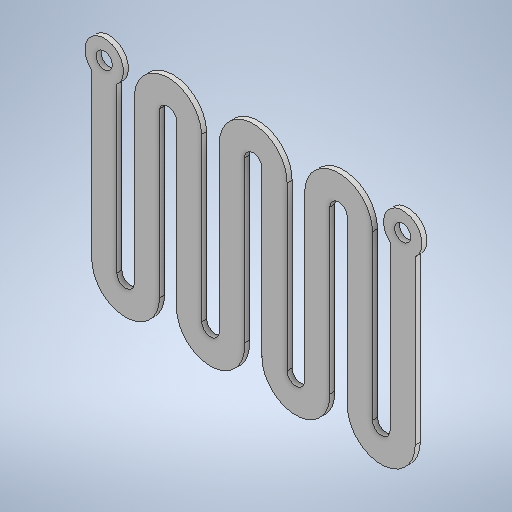
# Autodesk Inventor part: sensor2
Saved by Autodesk Inventor 2025.2 (Build 292293000, 293)
## iProperties
Created: 2025-01-22
Part Number: sensor2
Material: Generic
Document SubType Name: Modeling
Designer: Tony Dias
Density: 1 g/cm^3
Appearance: Default
Author: Tony Dias
Autodesk Inventor part; units mm, degrees
ref_plane "YZ Plane" through (0, 0, 0) normal (1, 0, 0) x (0, 1, 0)
ref_plane "XZ Plane" through (0, 0, 0) normal (0, 1, 0) x (-1, 0, 0)
ref_plane "XY Plane" through (0, 0, 0) normal (0, 0, 1) x (1, 0, 0)
sketch "Sketch1" plane through (0, 0, 0) normal (0, 0, 1) x (1, 0, 0)
  circle A0 centre (-59.5535, 47.2459) radius 7.653
  line L0 (-64.5524, 41.4512) -> (-64.5524, -23.1778)
  line L1 (-54.5526, 41.4529) -> (-54.5526, -23.5479)
  arc A1 (-54.5526, -23.5479) -> (-47.5527, -23.4962) centre (-51.0525, -23.5479) ccw
  line L2 (-47.5527, -23.4962) -> (-47.5527, 41.452)
  line L3 (-37.5474, 41.5644) -> (-37.5474, -23.5532)
  arc A2 (-64.5524, -23.1778) -> (-37.5474, -23.5515) centre (-51.0525, -23.5479) ccw
  arc A3 (-30.8632, 41.7144) -> (-37.5474, 41.5644) centre (-34.182, 40.6024) ccw
  line L4 (-30.8632, 41.7144) -> (-30.8632, -23.4297)
  line L5 (-20.7948, 41.1318) -> (-20.7948, -23.4297)
  arc A4 (-20.7947, 41.1274) -> (-47.5527, 41.452) centre (-34.182, 40.6024) ccw
  line L6 (-13.7626, 41.5703) -> (-13.7626, -23.4297)
  arc A5 (-20.7948, -23.4297) -> (-13.7626, -23.4297) centre (-17.2787, -23.4297) ccw
  line L7 (-3.7454, 41.5703) -> (-3.7454, -22.2525)
  arc A6 (-30.8632, -23.4297) -> (-3.7454, -22.2525) centre (-17.2787, -23.4297) ccw
  line L8 (3.17, 41.5703) -> (3.17, -23.406)
  line L9 (13.1831, 41.5703) -> (13.1831, -23.4297)
  arc A7 (3.17, 41.5703) -> (-3.7454, 41.5703) centre (-0.2877, 41.5703) ccw
  arc A8 (13.1831, 41.2384) -> (-13.7626, 41.5703) centre (-0.2877, 41.5703) ccw
  line L10 (20.1776, 41.5703) -> (20.1776, -23.4297)
  arc A9 (13.1831, -23.4297) -> (20.1776, -23.4297) centre (16.6804, -23.4297) ccw
  line L11 (30.1804, -22.8989) -> (30.1804, 41.5703)
  arc A10 (3.17, -23.406) -> (30.1804, -22.8989) centre (16.6804, -23.4297) ccw
  line L12 (37.1748, 41.5703) -> (37.1748, -23.4297)
  line L13 (47.1776, 41.5703) -> (47.1776, -23.4297)
  arc A11 (37.1748, 41.5703) -> (30.1804, 41.5703) centre (33.6776, 41.5703) ccw
  arc A12 (47.1776, 41.5703) -> (20.1776, 41.5703) centre (33.6776, 41.5703) ccw
  circle A13 centre (-59.5535, 47.2459) radius 3.25
  line L14 (54.172, -23.4297) -> (54.172, 41.4793)
  line L15 (64.1748, 41.4275) -> (64.1748, -23.4297)
  arc A14 (47.1776, -23.4297) -> (54.172, -23.4297) centre (50.6748, -23.4297) ccw
  arc A15 (37.1748, -23.4297) -> (64.1748, -23.4297) centre (50.6748, -23.4297) ccw
  circle A16 centre (59.2034, 47.2459) radius 7.653
  circle A17 centre (59.2034, 47.2459) radius 3.25
  point P0 (0, 0)
  point P1 (-51.0266, -27.048)
  point P2 (-51.2393, -37.0517)
  constraints: 36 point on circle, 32 end point, 18 centre point, 16 vertical, 11 tangent, 9 coincident, 1 point on line
extrude "Extrusion1" add sketch "Sketch1" along normal mid plane 2
body "Solid1"
